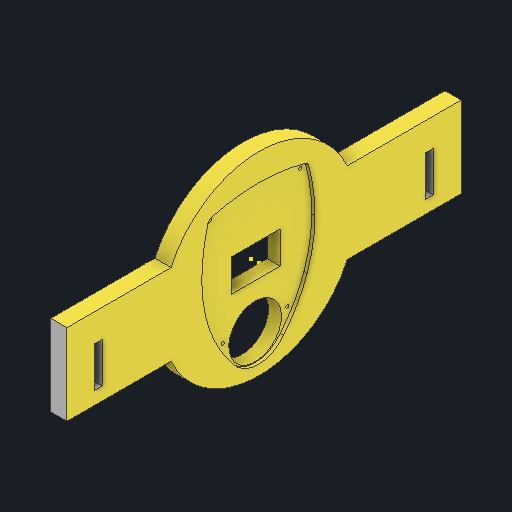
# Autodesk Inventor part: lidarholder
Saved by Autodesk Inventor 2027 (Build 310192000, 192)
## iProperties
Created: 2026-07-13
Part Number: lidarholder
Material: Generic
Document SubType Name: Modeling
Designer: uchiha
Density: 1 g/cm^3
Appearance: Default
Author: uchiha
Autodesk Inventor part; units mm, degrees
ref_plane "YZ Plane" through (0, 0, 0) normal (1, 0, 0) x (0, 1, 0)
ref_plane "XZ Plane" through (0, 0, 0) normal (0, 1, 0) x (-1, 0, 0)
ref_plane "XY Plane" through (0, 0, 0) normal (0, 0, 1) x (1, 0, 0)
sketch "Sketch1" plane through (0, 0, 0) normal (1, 0, 0) x (0, 1, 0)
  line L0 (-25.7214, 102.1584) -> (24.7536, 102.1584)
  line L1 (-25.7214, 76.1326) -> (-25.7214, 102.1584)
  line L2 (-25.7214, 76.1326) -> (-25.2196, 76.1326)
  line L3 (-25.2196, 76.1326) -> (-25.2196, 54.4992)
  arc A0 (-25.2196, 54.4992) -> (-25.2196, -54.5879) centre (-0.2196, -0.0444) ccw
  line L4 (-25.2196, -54.5879) -> (-25.2196, -76.2213)
  line L5 (-25.2028, -76.2213) -> (-25.2196, -76.2213)
  line L6 (-25.2028, -102.2471) -> (-25.2028, -76.2213)
  line L7 (24.9347, -102.2471) -> (-25.2028, -102.2471)
  line L8 (24.9347, -76.2213) -> (24.9347, -102.2471)
  line L9 (24.9347, -76.2213) -> (24.9615, -76.2213)
  line L10 (24.9615, -76.2213) -> (24.9615, -54.5879)
  arc A1 (24.9615, -54.5879) -> (24.9615, 54.4992) centre (-0.0385, -0.0444) ccw
  line L11 (24.9615, 54.4992) -> (24.9615, 76.1326)
  line L12 (24.9615, 76.1326) -> (24.7536, 76.1326)
  line L13 (24.7536, 102.1584) -> (24.7536, 76.1326)
  line L14 (24.9347, -107.2471) -> (24.9347, -102.2471)
  line L15 (24.9347, -102.2471) -> (-25.2028, -102.2471)
  line L16 (-25.2028, -102.2471) -> (-25.2028, -107.2471)
  line L17 (-25.2028, -107.2471) -> (24.9347, -107.2471)
  line L18 (24.7536, 102.1584) -> (24.7536, 107.1584)
  line L19 (24.7536, 107.1584) -> (-25.7214, 107.1584)
  line L20 (-25.7214, 107.1584) -> (-25.7214, 102.1584)
  line L21 (-25.7214, 102.1584) -> (24.7536, 102.1584)
  circle A2 centre (-33.7632, -19.5346) radius 1
  circle A3 centre (-33.7632, 20.4654) radius 1
  circle A4 centre (36.2368, -27.5346) radius 1
  circle A5 centre (36.2368, 28.4654) radius 1
  arc A6 (8.2368, -34.5346) -> (37.092, -30.6701) centre (8.2368, 75.1237) ccw
  arc A7 (37.092, -30.6701) -> (39.3723, -28.3898) centre (36.2368, -27.5346) ccw
  arc A8 (39.3723, -28.3898) -> (39.3723, 29.3206) centre (-66.4215, 0.4654) ccw
  arc A9 (39.3723, 29.3206) -> (37.092, 31.6009) centre (36.2368, 28.4654) ccw
  arc A10 (37.092, 31.6009) -> (8.2368, 35.4654) centre (8.2368, -74.1929) ccw
  arc A11 (8.2368, 35.4654) -> (-20.3455, 30.6591) centre (8.2368, -51.9243) ccw
  arc A12 (-20.3455, 30.6591) -> (-46.1402, 15.9514) centre (8.2368, -49.4429) ccw
  arc A13 (-46.1402, 15.9514) -> (-46.1402, -15.0206) centre (-34.7613, 0.4654) ccw
  arc A14 (-46.1402, -15.0206) -> (-20.3455, -29.7283) centre (8.2368, 50.3737) ccw
  arc A15 (-20.3455, -29.7283) -> (8.2368, -34.5346) centre (8.2368, 52.8551) ccw
  circle A16 centre (-37.2632, 0.4654) radius 16.3157
  point P0 (49.5286, -0.0444)
  point P1 (41.0675, 126.9871)
  point P2 (55.6621, 2.2018)
  dimension "d0" = 52.6592
  constraints: 44 end point, 24 point on circle, 17 centre point, 6 collinear
  measures "d0" distance of L10.end L14.start
extrude "Extrusion1" add sketch "Sketch1" along normal blind 10 contours L0 L13 L12 L11 A1 L10 L9 L8 L7 L6 L5 L4 A0 L3 L2 L1
extrude "Extrusion2" add sketch "Sketch1" along normal blind 8 contours A15 A14 A13 A12 A11 A10 A9 A8 A7 A6
extrude "Extrusion3" add sketch "Sketch1" along normal blind 10 and the other way blind 44.75 contours L20 L19 L18 L0 | L7 L14 L17 L16
sketch "Sketch2" plane through (10, 24.9347, -107.2471) normal (0, 0, -1) x (-1, 0, 0)
  circle A0 centre (42.75, -15) radius 1.5
  circle A1 centre (42.75, -35.1376) radius 1.5
  line L0 (54.75, -50.1376) -> (0, -50.1376) projected
  line L1 (54.75, 0) -> (0, 0) projected
  line L2 (54.75, 0) -> (54.75, -50.1376) projected
  point P0 (10, -24.9347)
  dimension "d9" = 3
  dimension "d10" = 3
  dimension "d11" = 15
  dimension "d12" = 15
  dimension "d13" = 12
  dimension "d14" = 12
  constraints: 2 centre point
  measures "d9" diameter of A0
  measures "d10" diameter of A1
  measures "d11" distance from line of L0 A1.centre
  measures "d12" distance from line of L1 A0.centre
  measures "d13" distance from line of L2 A0.centre
  measures "d14" distance from line of L2 A1.centre
extrude "Extrusion4" cut sketch "Sketch2" against normal blind 300
sketch "Sketch3" plane through (8, 0, 0) normal (1, 0, 0) x (0, 0, -1)
  line L0 (-15, -10) -> (15, -10)
  line L1 (15, -10) -> (15, 10)
  line L2 (15, 10) -> (-15, 10)
  line L3 (-15, 10) -> (-15, -10)
  line L4 (-15, -10) -> (15, 10) construction
  line L5 (15, -10) -> (-15, 10) construction
  point P0 (0, 0)
  dimension "d18" = 30
  dimension "d19" = 20
  constraints: 12 end point, 2 midpoint, 2 parallel, 1 horizontal, 1 perpendicular
  measures "d18" distance of L2.end L1.end
  measures "d19" distance of L1.end L0.end
extrude "Extrusion5" cut sketch "Sketch3" against normal blind 10
sketch "Sketch4" plane through (0, 24.9347, -76.2213) normal (0, 1, 0) x (1, 0, 0)
  point P0 (0, -76.2213)
sketch "Sketch5" plane through (10, 0, 0) normal (1, 0, 0) x (0, 0, -1)
  line L0 (102.2471, -25.2028) -> (102.2471, 24.9347) projected
  line L1 (107.2471, -25.2028) -> (107.2471, 24.9347) projected
  line L2 (102.2471, -25.2028) -> (107.2471, -25.2028)
  line L3 (107.2471, -25.2028) -> (107.2471, 24.9347)
  line L4 (107.2471, 24.9347) -> (102.2471, 24.9347)
  line L5 (102.2471, 24.9347) -> (102.2471, -25.2028)
  line L6 (76.2213, -25.2028) -> (107.2471, -25.2028) projected
  line L7 (102.2471, 12.5969) -> (107.2471, 12.5969)
  line L8 (107.2471, 12.5969) -> (107.2471, -12.4031)
  line L9 (107.2471, -12.4031) -> (102.2471, -12.4031)
  line L10 (102.2471, -12.4031) -> (102.2471, 12.5969)
  line L11 (102.2471, 12.5969) -> (107.2471, -12.4031) construction
  line L12 (107.2471, 12.5969) -> (102.2471, -12.4031) construction
  line L13 (107.2471, -25.2028) -> (117.2471, -25.2028)
  line L14 (117.2471, -25.2028) -> (117.2471, 24.9347)
  line L15 (117.2471, 24.9347) -> (107.2471, 24.9347)
  line L16 (107.2471, 24.9347) -> (107.2471, -25.2028)
  line L17 (0, 0) -> (0, -27.4192)
  line L18 (-102.2471, 12.5969) -> (-107.2471, 12.5969)
  line L19 (-107.2471, 12.5969) -> (-107.2471, -12.4031)
  line L20 (-107.2471, -12.4031) -> (-102.2471, -12.4031)
  line L21 (-102.2471, -12.4031) -> (-102.2471, 12.5969)
  line L22 (-102.2471, 12.5969) -> (-107.2471, -12.4031) construction
  line L23 (-107.2471, 12.5969) -> (-102.2471, -12.4031) construction
  point P0 (104.7471, 0.0969)
  point P1 (104.7471, -12.4031)
  point P2 (-104.7471, 0.0969)
  point P3 (-104.7471, -12.4031)
  dimension "d22" = 5
  dimension "d24" = 12.5
  dimension "d25" = 5
  dimension "d27" = 10
  constraints: 42 end point, 6 parallel, 6 symmetric about line, 3 horizontal, 3 midpoint, 3 perpendicular, 2 collinear, 1 vertical
  measures "d22" distance of L8.end L9.end
  measures "d24" distance of point (104.747, -12.403) point (104.747, 0.097)
  measures "d25" distance between parallel lines of L0 L1
  measures "d27" distance of L15.end L14.end
extrude "Extrusion6" add sketch "Sketch5" against normal blind 10 contours L1 L15 L14 L13
extrude "Extrusion7" cut sketch "Sketch5" against normal blind 10 contours L0 L7 L1 L9
ref_plane "Work Plane1" through (0, 24.9347, -76.2213) normal (0, 1, 0) x (1, 0, 0)
sketch "Sketch6" plane through (0, 24.9347, -76.2213) normal (0, 1, 0) x (1, 0, 0)
  point P0 (0, -76.2213)
sketch "Sketch7" plane through (0, 24.9347, -76.2213) normal (0, 1, 0) x (1, 0, 0)
  line L0 (-44.75, 31.0258) -> (0, 31.0258) projected
  line L1 (0, 26.0258) -> (-44.75, 26.0258) projected
  line L2 (-44.75, 26.0258) -> (-44.75, 31.0258) projected
  line L3 (10, 31.0258) -> (0, 31.0258) projected
  line L4 (0, 26.0258) -> (0, 31.0258) projected
  line L5 (10, 26.0258) -> (10, 31.0258) projected
  line L6 (10, 26.0258) -> (0, 26.0258) projected
  line L7 (0, 41.0258) -> (0, 31.0258) projected
  line L8 (0, 31.0258) -> (0, 41.0258) projected
  line L9 (10, 26.0258) -> (0, 26.0258) projected
  line L10 (10, 41.0258) -> (0, 41.0258) projected
  line L11 (10, 31.0258) -> (10, 26.0258) projected
  line L12 (10, 31.0258) -> (0, 31.0258) projected
  line L13 (0, 31.0258) -> (0, 26.0258) projected
  line L14 (10, 41.0258) -> (0, 41.0258) projected
  line L15 (-44.75, 26.0258) -> (0, 26.0258) projected
  line L16 (-44.75, 31.0258) -> (0, 31.0258) projected
  line L17 (-44.75, 31.0258) -> (-44.75, 26.0258) projected
  line L18 (-34.25, 31.0258) -> (-31.25, 31.0258) projected
  line L19 (-31.25, 26.0258) -> (-34.25, 26.0258) projected
  line L20 (-34.25, 31.0258) -> (-31.25, 31.0258) projected
  line L21 (-31.25, 26.0258) -> (-34.25, 26.0258) projected
  line L22 (10, 26.0258) -> (0, 26.0258) projected
  line L23 (10, 26.0258) -> (0, 26.0258) projected
  line L24 (10, 26.0258) -> (10, 31.0258) projected
  line L25 (10, 26.0258) -> (0, 26.0258) projected
  line L26 (0, 26.0258) -> (0, 31.0258) projected
  line L27 (10, 31.0258) -> (0, 31.0258) projected
  line L28 (10, 31.0258) -> (0, 31.0258) projected
  line L29 (10, 31.0258) -> (0, 31.0258) projected
  line L30 (10, 31.0258) -> (10, 26.0258) projected
  line L31 (10, 31.0258) -> (0, 31.0258) projected
  line L32 (0, 31.0258) -> (0, 26.0258) projected
  line L33 (10, 26.0258) -> (0, 26.0258) projected
  line L34 (-31.25, 26.0258) -> (-34.25, 26.0258) projected
  line L35 (-34.25, 31.0258) -> (-31.25, 31.0258) projected
  line L36 (-31.25, 26.0258) -> (-34.25, 26.0258) projected
  line L37 (-34.25, 31.0258) -> (-31.25, 31.0258) projected
  line L38 (-31.25, 26.0258) -> (-34.25, 26.0258) projected
  line L39 (-31.25, 26.0258) -> (-34.25, 26.0258) projected
  line L40 (0, 26.0258) -> (-44.75, 26.0258) projected
  line L41 (-44.75, 26.0258) -> (0, 26.0258) projected
  line L42 (-44.75, 31.0258) -> (0, 31.0258) projected
  line L43 (-44.75, 31.0258) -> (0, 31.0258) projected
  line L44 (-34.25, 31.0258) -> (-31.25, 31.0258) projected
  line L45 (-34.25, 31.0258) -> (-31.25, 31.0258) projected
  line L46 (-44.75, 26.0258) -> (-44.75, 31.0258) projected
  line L47 (-44.75, 31.0258) -> (-44.75, 26.0258) projected
  line L48 (10, 41.0258) -> (0, 41.0258) projected
  line L49 (10, 41.0258) -> (0, 41.0258) projected
  line L50 (0, 31.0258) -> (0, 41.0258) projected
  line L51 (0, 41.0258) -> (0, 31.0258) projected
  line L52 (0, 26.0258) -> (0, 31.0258) projected
  line L53 (0, 31.0258) -> (0, 26.0258) projected
  line L54 (-44.75, 31.0258) -> (10, 31.0258) projected
  line L55 (-44.75, 31.0258) -> (10, 31.0258) projected
  line L56 (10, 31.0258) -> (10, 26.0258) projected
  line L57 (10, 26.0258) -> (-44.75, 26.0258) projected
  line L58 (-44.75, 26.0258) -> (-44.75, 31.0258) projected
  line L59 (0, 26.0258) -> (-44.75, 26.0258) projected
  line L60 (0, 26.0258) -> (0, 0) projected
  line L61 (0, 0) -> (10, 0) projected
  line L62 (10, 41.0258) -> (10, 0) projected
  line L63 (10, 41.0258) -> (0, 41.0258) projected
  line L64 (0, 31.0258) -> (0, 41.0258) projected
  line L65 (-44.75, 31.0258) -> (0, 31.0258) projected
  line L66 (-44.75, 26.0258) -> (-44.75, 31.0258) projected
  line L67 (0, 26.0258) -> (-44.75, 26.0258) projected
  line L68 (0, 31.0258) -> (0, 26.0258)
  point P0 (0, -76.2213)
  constraints: 2 end point, 1 collinear, 6 other
extrude "Extrusion8" cut sketch "Sketch7" against normal blind 100 contours L0 L4 L1 L2
sketch "Sketch8" plane through (0, 24.9347, -76.2213) normal (0, 1, 0) x (1, 0, 0)
  line L0 (10, 26.0258) -> (-44.75, 26.0258) projected
  line L1 (-44.75, 31.0258) -> (10, 31.0258) projected
  line L2 (-44.75, 26.0258) -> (10, 26.0258)
  line L3 (10, 26.0258) -> (10, 31.0258)
  line L4 (10, 31.0258) -> (-44.75, 31.0258)
  line L5 (-44.75, 31.0258) -> (-44.75, 26.0258)
  point P0 (0, -76.2213)
  constraints: 8 end point, 2 parallel, 1 horizontal, 1 perpendicular
sketch "Sketch9" plane through (0, 24.7536, 76.1326) normal (0, 1, 0) x (1, 0, 0)
  line L0 (0, 0) -> (0, -26.0258) projected
  line L1 (10, -31.0258) -> (-44.75, -31.0258) projected
  line L2 (0, -26.0258) -> (-44.75, -26.0258)
  line L3 (-44.75, -26.0258) -> (-44.75, -31.0258)
  line L4 (-44.75, -31.0258) -> (0, -31.0258)
  line L5 (0, -31.0258) -> (0, -26.0258)
  point P0 (0, 76.1326)
  constraints: 8 end point, 2 parallel, 1 horizontal, 1 perpendicular
extrude "Extrusion9" cut sketch "Sketch9" against normal blind 100
sketch "Sketch10" plane through (10, 0, 0) normal (1, 0, 0) x (0, 0, -1)
  line L0 (-107.1584, 24.7536) -> (-107.1584, -25.7214) projected
  line L1 (-107.1584, -25.7214) -> (-117.1584, -25.7214)
  line L2 (-117.1584, -25.7214) -> (-117.1584, 24.7536)
  line L3 (-117.1584, 24.7536) -> (-107.1584, 24.7536)
  line L4 (-107.1584, 24.7536) -> (-107.1584, -25.7214)
  point P0 (0, 0)
  dimension "d37" = 10
  constraints: 8 end point, 2 parallel, 1 horizontal, 1 perpendicular
  measures "d37" distance of L2.end L3.end
extrude "Extrusion10" add sketch "Sketch10" against normal blind 10
extrude "Extrusion11" cut sketch "Sketch5" against normal up to next contours L21 L20 L19 L18
sketch "Sketch11" plane through (10, 0, 0) normal (1, 0, 0) x (0, 0, -1)
  line L0 (107.2471, 12.5969) -> (107.2471, -12.4031) projected
  line L1 (102.2471, -12.4031) -> (102.2471, 12.5969) projected
  line L2 (102.2471, 12.5969) -> (107.2471, 12.5969) projected
  line L3 (107.2471, -12.4031) -> (102.2471, -12.4031) projected
  line L4 (97.8301, 12.5969) -> (97.8301, -12.4031)
  line L5 (92.8301, -12.4031) -> (92.8301, 12.5969)
  line L6 (92.8301, 12.5969) -> (97.8301, 12.5969)
  line L7 (97.8301, -12.4031) -> (92.8301, -12.4031)
  point P0 (0, 0)
  point P1 (39.1416, -10.1412)
  dimension "d43" = 4.417
  dimension "d48" = 25
  dimension "d49" = 5
  constraints: 8 end point, 1 collinear
  measures "d43" distance between parallel lines of L4 L1
  measures "d48" distance of L5.start L5.end
  measures "d49" distance of L5.end L4.start
extrude "Extrusion12" cut sketch "Sketch11" against normal blind 10 contours L4 L7 L5 L6
extrude "Extrusion13" add sketch "Sketch11" against normal blind 10 contours L0 L3 L1 L2
ref_plane "Work Plane2" through (5, 0, 0) normal (1, 0, 0) x (0, 0, -1)
sketch "Sketch12" plane through (10, 0, 0) normal (1, 0, 0) x (0, 0, -1)
  point P0 (0, 0)
sketch "Sketch13" plane through (10, 0, 0) normal (1, 0, 0) x (0, 0, -1)
  line L0 (-102.2471, -12.4031) -> (-107.2471, -12.4031) projected
  line L1 (-102.2471, 12.5969) -> (-102.2471, -12.4031) projected
  line L2 (-107.2471, -12.4031) -> (-107.2471, 12.5969) projected
  line L3 (-107.2471, 12.5969) -> (-102.2471, 12.5969) projected
  point P0 (0, 0)
extrude "Extrusion14" add sketch "Sketch13" against normal blind 10
sketch "Sketch14" plane through (5, 0, 0) normal (1, 0, 0) x (0, 0, -1)
  point P0 (0, 0)
sketch "Sketch15" plane through (10, 0, 0) normal (1, 0, 0) x (0, 0, -1)
  line L0 (0, 0) -> (0, 38.3615)
  line L1 (92.8301, -12.4031) -> (92.8301, 12.5969) projected
  line L2 (97.8301, 12.5969) -> (97.8301, -12.4031) projected
  line L3 (97.8301, -12.4031) -> (92.8301, -12.4031) projected
  line L4 (92.8301, 12.5969) -> (97.8301, 12.5969) projected
  line L5 (-107.1699, -12.4031) -> (-112.1699, -12.4031)
  line L6 (-112.1699, -12.4031) -> (-112.1699, 12.5969)
  line L7 (-112.1699, 12.5969) -> (-107.1699, 12.5969)
  line L8 (-107.1699, 12.5969) -> (-107.1699, -12.4031)
  dimension "d53" = 5
  dimension "d54" = 200
  constraints: 10 end point, 2 parallel, 1 horizontal, 1 perpendicular, 1 vertical
  measures "d53" distance of L6.end L7.end
  measures "d54" distance between parallel lines of L8 L1
extrude "Extrusion15" cut sketch "Sketch15" against normal blind 10 contours L5 L6 L7 L8
sketch "Sketch16" plane through (10, 0, 0) normal (1, 0, 0) x (0, 0, -1)
  point P0 (0, 0)
sketch "Sketch17" plane through (10, 0, 0) normal (1, 0, 0) x (0, 0, -1)
  line L0 (-117.1584, -25.7214) -> (-76.1326, -25.7214) projected
  line L1 (-117.1584, -25.7214) -> (-128.7644, -25.7214)
  line L2 (-128.7644, -25.7214) -> (-128.7644, 24.4286)
  line L3 (-128.7644, 24.4286) -> (-117.1584, 24.4286)
  line L4 (-117.1584, 24.4286) -> (-117.1584, -25.7214)
  line L5 (-76.1326, -25.2196) -> (-54.4992, -25.2196) projected
  line L6 (117.2471, -25.2028) -> (117.2471, 24.9347) projected
  point P0 (0, 0)
  dimension "d58" = 117.2471
  dimension "d59" = 128.7644
  dimension "d60" = 11.606
  constraints: 8 end point, 2 parallel, 1 horizontal, 1 perpendicular
  measures "d58" distance from line of point (0, 0) L6
  measures "d59" distance from line of L2 point (0, 0)
  measures "d60" distance of L2.end L3.end
extrude "Extrusion16" add sketch "Sketch17" against normal blind 10
sketch "Sketch18" plane through (10, 0, 0) normal (1, 0, 0) x (0, 0, -1)
  circle A0 centre (0, 0) radius 59.9998
  line L0 (117.2471, -25.2028) -> (117.2471, 24.9347) projected
  line L1 (76.2213, -25.2028) -> (117.2471, -25.2028) projected
  line L2 (54.5879, -25.2196) -> (76.2213, -25.2196) projected
  line L3 (76.2213, 24.9615) -> (54.5879, 24.9615) projected
  line L4 (117.2471, 24.9347) -> (76.2213, 24.9347) projected
  line L5 (76.2213, -25.2196) -> (117.2639, -25.2196)
  line L6 (117.2639, -25.2196) -> (117.2639, 24.9515)
  line L7 (117.2639, 24.9515) -> (76.2213, 24.9515)
  line L8 (54.5879, -25.2196) -> (76.2213, -25.2196)
  line L9 (117.2639, -25.2196) -> (59.9998, -25.2196)
  line L10 (59.9998, -25.2196) -> (59.9998, 24.9615)
  line L11 (59.9998, 24.9615) -> (117.2639, 24.9615)
  line L12 (117.2639, 24.9615) -> (117.2639, -25.2196)
  line L13 (-59.9998, -24.9615) -> (-59.9998, 24.9615)
  line L14 (-128.7644, -25.7214) -> (-76.1326, -25.7214) projected
  line L15 (-59.9998, 24.9615) -> (-128.7644, 24.9615)
  line L16 (-128.7644, 24.9615) -> (-128.7644, -25.7214)
  line L17 (-128.7644, -25.7214) -> (-59.9998, -25.7214)
  line L18 (-59.9998, -25.7214) -> (-59.9998, 24.9615)
  constraints: 26 end point, 5 equal length, 2 horizontal, 2 perpendicular, 1 centre point, 1 coincident, 1 point on line, 1 tangent, 2 other
extrude "Extrusion17" cut sketch "Sketch18" against normal blind 10 contours L13 L18 L17 L14 L16 L15 | L10 L3 L11 L12 L6 L5 L2
sketch "Sketch19" plane through (10, -25.2196, -59.9998) normal (0, 0, -1) x (-1, 0, 0)
  line L0 (0, 0) -> (0, 50.1811) projected
  line L1 (10, 0) -> (0, 0) projected
  line L2 (10, 50.1811) -> (10, 0) projected
  line L3 (0, 50.1811) -> (10, 50.1811) projected
  point P0 (10, 25.2196)
extrude "Extrusion18" add sketch "Sketch19" along normal blind 65
sketch "Sketch20" plane through (10, -25.2196, 59.9998) normal (0, 0, 1) x (1, 0, 0)
  point P0 (-10, 25.2196)
sketch "Sketch21" plane through (10, -25.2196, 59.9998) normal (0, 0, 1) x (1, 0, 0)
  point P0 (-10, 25.2196)
sketch "Sketch22" plane through (0, 0, 0) normal (-1, 0, 0) x (0, 0, 1)
  line L0 (59.9998, 24.9615) -> (59.9998, -25.2196) projected
  line L1 (59.9998, -25.2196) -> (59.9998, 24.9615) projected
sketch "Sketch23" plane through (10, -25.2196, 59.9998) normal (0, 0, 1) x (1, 0, 0)
  line L0 (0, 0) -> (-10, 0) projected
  line L1 (0, 50.1811) -> (0, 0) projected
  line L2 (-10, 50.1811) -> (0, 50.1811) projected
  line L3 (-10, 0) -> (-10, 50.1811) projected
  point P0 (-10, 25.2196)
extrude "Extrusion19" add sketch "Sketch23" along normal blind 70
sketch "Sketch24" plane through (0, 0, 0) normal (-1, 0, 0) x (0, 0, 1)
  line L0 (-102.9957, 7.6613) -> (-107.7957, 7.6613)
  line L1 (-107.7957, 7.6613) -> (-107.7957, -17.1387)
  line L2 (-107.7957, -17.1387) -> (-102.9957, -17.1387)
  line L3 (-102.9957, -17.1387) -> (-102.9957, 7.6613)
  line L4 (-102.9957, 7.6613) -> (-107.7957, -17.1387) construction
  line L5 (-107.7957, 7.6613) -> (-102.9957, -17.1387) construction
  line L6 (101.8043, 7.6613) -> (97.0043, 7.6613)
  line L7 (97.0043, 7.6613) -> (97.0043, -17.1387)
  line L8 (97.0043, -17.1387) -> (101.8043, -17.1387)
  line L9 (101.8043, -17.1387) -> (101.8043, 7.6613)
  line L10 (101.8043, 7.6613) -> (97.0043, -17.1387) construction
  line L11 (97.0043, 7.6613) -> (101.8043, -17.1387) construction
  line L12 (-124.9998, -25.2196) -> (-124.9998, 24.9615) projected
  point P0 (0, 0)
  point P1 (-105.3957, -4.7387)
  point P2 (99.4043, -4.7387)
  dimension "d69" = 200
  dimension "d70" = 4.8
  dimension "d71" = 17.2041
  dimension "d75" = 24.8
  constraints: 24 end point, 4 midpoint, 4 parallel, 2 equal length, 2 horizontal, 2 perpendicular, 1 point on line
  measures "d69" distance between parallel lines of L7 L3
  measures "d70" distance of L7.end L8.end
  measures "d71" distance between parallel lines of L12 L1
  measures "d75" distance of L2.end L0.start
extrude "Extrusion20" cut sketch "Sketch24" against normal blind 70
ref_plane "Work Plane3" through (5, 0, 0) normal (-1, 0, 0) x (0, 0, 1)
sketch "Sketch26" plane through (10, 0, 0) normal (1, 0, 0) x (0, 0, -1)
  line L0 (-129.9998, -25.2196) -> (-129.9998, 24.9615) projected
  line L1 (-129.9998, 24.9615) -> (-118.8443, 24.9615)
  line L2 (-118.8443, 24.9615) -> (-118.8443, -25.2196)
  line L3 (-118.8443, -25.2196) -> (-129.9998, -25.2196)
  line L4 (-129.9998, -25.2196) -> (-129.9998, 24.9615)
  line L5 (-101.8043, -17.1387) -> (-101.8043, 7.6613) projected
  point P0 (0, 0)
  point P1 (-118.8443, -0.129)
  dimension "d77" = 17.04
  constraints: 8 end point, 2 parallel, 1 horizontal, 1 midpoint, 1 perpendicular
  measures "d77" distance from line of point (-118.844, -0.129) L5
extrude "Extrusion21" cut sketch "Sketch26" against normal blind 10
body "Solid1"
